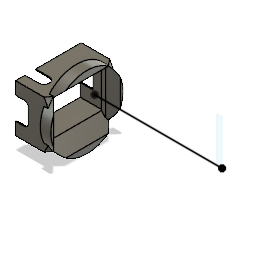
PS Vita Akaso Case v2 (Autodesk Fusion 360 design; units mm, degrees)
Autodesk Fusion 360 part; units mm, degrees
sketch "Sketch1" plane through (0, 0, 0) normal (1, 0, 0) x (0, 0, -1)
  line L0 (0, 0) -> (59, 0)
  line L1 (59, 0) -> (59, 42)
  line L2 (59, 42) -> (0, 42)
  line L3 (0, 42) -> (0, 0)
  line L4 (59, 42) -> (41.5, 42)
  line L5 (41.5, 42) -> (41.5, 24.5)
  line L6 (41.5, 24.5) -> (59, 24.5)
  line L7 (59, 24.5) -> (59, 42)
  circle A0 centre (41.5, 24.5) radius 10.5
  dimension "d1" = 59
  dimension "d2" = 42
  dimension "d3" = 17.5
  dimension "d4" = 17.5
  dimension "d5" = 21
  constraint horizontal L0
  constraint vertical L1
  constraint horizontal L2
  constraint vertical L3
  constraint coincident L0.start L3.end
  constraint horizontal L4
  constraint vertical L5
  constraint horizontal L6
  constraint vertical L7
  constraint coincident L5.end L6.start
  measures "d1" distance of L0.start L0.end
  measures "d2" distance of L0.start L2.end
  measures "d3" distance of L1.end L4.end
  measures "d4" distance of L1.end L6.end
  measures "d5" diameter of A0
extrude "Extrude1" add sketch "Sketch1" against normal blind 25 makes body 1
extrude "Extrude2" add sketch "Sketch1" along normal blind 5 contours L5 L6 A0 | L5 L6 A0 bodies 1
sketch "Sketch2" plane through (0, 0, 0) normal (1, 0, 0) x (0, 0, -1)
  line L0 (0, 0) -> (-182, 0)
  line L1 (0, 0) -> (-182, 0)
  line L2 (-182, 0) -> (-182, 84)
  line L3 (-182, 84) -> (0, 84)
  line L4 (0, 84) -> (0, 0)
  dimension "d10" = 182
  dimension "d11" = 182
  dimension "d12" = 84
  constraint coincident L0.start L1.start
  constraint horizontal L0
  constraint horizontal L1
  constraint vertical L2
  constraint horizontal L3
  constraint vertical L4
  measures "d10" distance of L0.start L0.end
  measures "d11" distance of L0.start L0.end
  measures "d12" distance of L0.start L3.end
extrude "Extrude3" add sketch "Sketch2" along normal blind 150 and the other way blind -132 separate body makes body 2
sketch "Sketch3" plane through (132, 0, 0) normal (-1, 0, 0) x (0, 0, 1)
  line L0 (182, 84) -> (0, 84)
  line L1 (0, 84) -> (0, 0)
  line L2 (0, 0) -> (182, 0)
  line L3 (182, 0) -> (182, 84)
  line L4 (0, 42) -> (182, 42)
  line L5 (91, 84) -> (91, 0)
  point P0 (0, 42)
  constraint coincident P0 L4.start
  constraint midpoint L3 L4.end
  constraint midpoint L0 L5.start
  constraint midpoint L2 L5.end
extrude "Extrude4" add sketch "Sketch3" along normal blind 5 contours L0 L3 L4 L5 bodies 2
sketch "Sketch4" plane through (0, 0, 91) normal (0, 0, -1) x (-1, 0, 0)
  line L0 (-132, 84) -> (-132, 42)
  line L1 (-132, 42) -> (-127, 42)
  line L2 (-127, 42) -> (-127, 84)
  line L3 (-127, 84) -> (-132, 84)
  line L4 (-132, 42) -> (-12, 42)
  dimension "d19" = 120
  constraint coincident L0.end L1.start
  constraint perpendicular L2 L4
  measures "d19" distance of L0.end L4.end
move_body "Move1" bodies 1 to x (1, 0, 0) y (0, 1, 0) z (0, 0, 1) at (-8.649, 1.2848, 93.06)
move_body "Move2" bodies 1 to x (1, 0, 0) y (0, 1, 0) z (0, 0, 1) at (15, 15, 40)
extrude "Extrude5" cut 1 faces at (127, 70, 121.3333) along direction (1, 0, 0) blind 5 on bodies 2 bodies 2
sketch "Sketch5" plane through (0, 0, 74.06) normal (0, 0, -1) x (-1, 0, 0)
  line L0 (-6.351, 58.2848) -> (-6.351, 16.2848)
  line L1 (-6.351, 16.2848) -> (18.649, 16.2848)
  line L2 (18.649, 16.2848) -> (18.649, 58.2848)
  line L3 (18.649, 58.2848) -> (-6.351, 58.2848)
  line L4 (-6.351, 58.2848) -> (-6.351, 58.7848)
  line L5 (-6.351, 58.7848) -> (-6.851, 58.7848)
  line L6 (-6.851, 58.7848) -> (19.149, 58.7848)
  line L7 (19.149, 58.7848) -> (19.149, 15.7848)
  line L8 (19.149, 15.7848) -> (-6.851, 15.7848)
  line L9 (-6.851, 15.7848) -> (-6.851, 58.7848)
  dimension "d22" = 0.5
  dimension "d23" = 0.5
  dimension "d24" = 43
  dimension "d25" = 26
  constraint coincident L0.start L3.end
  constraint vertical L4
  constraint perpendicular L4 L5
  constraint horizontal L6
  constraint vertical L7
  constraint horizontal L8
  constraint vertical L9
  measures "d22" distance of L0.start L4.end
  measures "d23" distance of L4.end L5.end
  measures "d24" distance of L5.end L8.end
  measures "d25" distance of L5.end L6.end
extrude "Extrude6" add sketch "Sketch5" along normal blind 2 and the other way blind -0.5 separate body makes body 3
sketch "Sketch6" plane through (0, 0, 72.06) normal (0, 0, -1) x (-1, 0, 0)
  line L0 (-6.351, 58.2848) -> (18.649, 58.2848)
  line L1 (18.649, 58.2848) -> (18.649, 16.2848)
  line L2 (18.649, 16.2848) -> (-6.351, 16.2848)
  line L3 (-6.351, 16.2848) -> (-6.351, 58.2848)
  line L4 (-6.851, 15.7848) -> (19.149, 15.7848)
  line L5 (19.149, 15.7848) -> (19.149, 58.7848)
  line L6 (19.149, 58.7848) -> (-6.851, 58.7848)
  line L7 (-6.851, 58.7848) -> (-6.851, 15.7848)
extrude "Extrude7" add sketch "Sketch6" against normal blind 0.5 contours L0 L1 L2 L3 bodies 3
extrude "Extrude8" add 1 faces at (-1.9824, 44.2848, 72.56) along direction (0, 0, 1) blind 1 on bodies 3 bodies 3
extrude "Extrude9" add 1 faces at (6.851, 30.1181, 73.06) along direction (1, 0, 0) blind 1 on bodies 3 bodies 3
sketch "Sketch7" plane through (0, 0, 73.56) normal (0, 0, 1) x (1, 0, 0)
  line L0 (-19.149, 15.7848) -> (7.851, 15.7848)
  line L1 (7.851, 15.7848) -> (7.851, 58.7848)
  line L2 (7.851, 58.7848) -> (-19.149, 58.7848)
  line L3 (-19.149, 58.7848) -> (-19.149, 15.7848)
  line L4 (7.851, 58.7848) -> (6.851, 58.7848)
  line L5 (6.851, 58.7848) -> (6.851, 15.7848)
  line L6 (6.851, 15.7848) -> (7.851, 15.7848)
  line L7 (7.851, 15.7848) -> (7.851, 58.7848)
  dimension "d36" = 1
  constraint horizontal L4
  constraint vertical L5
  constraint horizontal L6
  constraint vertical L7
  constraint coincident L1.end L2.start
  measures "d36" distance of L1.end L4.end
extrude "Extrude10" add sketch "Sketch7" along normal blind 6 contours L0 L1 L2 L4 L5 L6 L7 bodies 3
extrude "Extrude11" add 1 faces at (-1.4824, 58.7848, 72.56) along direction (0, 1, 0) blind 1 on bodies 3 bodies 3
sketch "Sketch8" plane through (0, 0, 73.56) normal (0, 0, 1) x (1, 0, 0)
  line L0 (6.851, 15.7848) -> (6.851, 59.7848)
  line L1 (6.851, 59.7848) -> (-19.149, 59.7848)
  line L2 (-19.149, 59.7848) -> (-19.149, 15.7848)
  line L3 (-19.149, 15.7848) -> (6.851, 15.7848)
  line L4 (6.851, 59.7848) -> (-19.149, 59.7848)
  line L5 (-19.149, 59.7848) -> (-19.149, 58.7848)
  line L6 (-19.149, 58.7848) -> (6.851, 58.7848)
  line L7 (6.851, 58.7848) -> (6.851, 59.7848)
  dimension "d41" = 1
  constraint horizontal L4
  constraint vertical L5
  constraint horizontal L6
  constraint vertical L7
  constraint coincident L0.end L1.start
  measures "d41" distance of L0.end L6.end
extrude "Extrude12" add sketch "Sketch8" along normal blind 61 contours L0 L1 L2 L4 L5 L6 L7 bodies 3
sketch "Sketch9" plane through (0, 58.7848, 0) normal (0, -1, 0) x (1, 0, 0)
  line L0 (-19.149, 73.56) -> (6.851, 73.56)
  line L1 (6.851, 73.56) -> (6.851, 79.56)
  line L2 (6.851, 79.56) -> (6.851, 134.56)
  line L3 (6.851, 134.56) -> (-19.149, 134.56)
  line L4 (-19.149, 134.56) -> (-19.149, 73.56)
  line L5 (-19.149, 134.56) -> (6.851, 134.56)
  line L6 (6.851, 134.56) -> (6.851, 133.56)
  line L7 (6.851, 133.56) -> (-19.149, 133.56)
  line L8 (-19.149, 133.56) -> (-19.149, 134.56)
  dimension "d44" = 1
  constraint horizontal L5
  constraint vertical L6
  constraint horizontal L7
  constraint vertical L8
  constraint coincident L3.end L4.start
  measures "d44" distance of L3.end L7.end
extrude "Extrude13" add sketch "Sketch9" along normal blind 44 contours L2 L3 L4 L5 L6 L7 L8 bodies 3
sketch "Sketch10" plane through (0, 0, 133.56) normal (0, 0, -1) x (-1, 0, 0)
  line L0 (19.149, 58.7848) -> (-6.851, 58.7848)
  line L1 (-6.851, 58.7848) -> (-6.851, 14.7848)
  line L2 (-6.851, 14.7848) -> (19.149, 14.7848)
  line L3 (19.149, 14.7848) -> (19.149, 58.7848)
  line L4 (19.149, 14.7848) -> (-6.851, 14.7848)
  line L5 (-6.851, 14.7848) -> (-6.851, 15.7848)
  line L6 (-6.851, 15.7848) -> (19.149, 15.7848)
  line L7 (19.149, 15.7848) -> (19.149, 14.7848)
  point P0 (-6.851, 15.7848)
  constraint horizontal L4
  constraint vertical L5
  constraint horizontal L6
  constraint vertical L7
  constraint coincident P0 L5.end
  constraint coincident L2.end L3.start
extrude "Extrude14" add 1 faces at (-1.4824, 15.7848, 72.56) along direction (0, -1, 0) blind 1 on bodies 3 bodies 3
extrude "Extrude15" add sketch "Sketch10" along normal blind 60 contours L1 L2 L3 L4 L5 L6 L7 bodies 3
extrude "Extrude16" add 1 faces at (6.851, 15.1181, 115.8933) along direction (1, 0, 0) blind 1 on bodies 3 bodies 3
sketch "Sketch11" plane through (0, 0, 133.56) normal (0, 0, -1) x (-1, 0, 0)
  line L0 (-7.851, 15.7848) -> (19.149, 15.7848)
  line L1 (19.149, 15.7848) -> (19.149, 58.7848)
  line L2 (19.149, 58.7848) -> (-7.851, 58.7848)
  line L3 (-7.851, 58.7848) -> (-7.851, 15.7848)
  line L4 (-7.851, 15.7848) -> (-6.851, 15.7848)
  line L5 (-6.851, 15.7848) -> (-6.851, 58.7848)
  line L6 (-6.851, 58.7848) -> (-7.851, 58.7848)
  line L7 (-7.851, 58.7848) -> (-7.851, 15.7848)
  dimension "d53" = 1
  constraint horizontal L4
  constraint vertical L5
  constraint horizontal L6
  constraint vertical L7
  constraint coincident L0.start L3.end
  measures "d53" distance of L0.start L4.end
extrude "Extrude17" add sketch "Sketch11" along normal blind 5 contours L0 L2 L3 L4 L5 L6 L7 bodies 3
sketch "Sketch12" plane through (0, 58.7848, 0) normal (0, -1, 0) x (1, 0, 0)
  line L0 (7.851, 128.56) -> (6.851, 128.56)
  line L1 (6.851, 128.56) -> (6.851, 133.56)
  line L2 (6.851, 133.56) -> (-19.149, 133.56)
  line L3 (-19.149, 133.56) -> (-19.149, 73.56)
  line L4 (-19.149, 73.56) -> (6.851, 73.56)
  line L5 (6.851, 73.56) -> (6.851, 79.56)
  line L6 (6.851, 79.56) -> (7.851, 79.56)
  line L7 (7.851, 79.56) -> (7.851, 128.56)
  line L8 (7.851, 128.56) -> (6.851, 128.56)
  line L9 (6.851, 128.56) -> (6.851, 79.56)
  line L10 (6.851, 79.56) -> (7.851, 79.56)
  line L11 (7.851, 79.56) -> (7.851, 128.56)
  constraint horizontal L8
  constraint vertical L9
  constraint horizontal L10
  constraint vertical L11
  constraint coincident L5.end L6.start
  constraint coincident L0.start L7.end
extrude "Extrude18" add sketch "Sketch12" along normal blind 5 contours L0 L6 L7 L8 L9 L10 L11 bodies 3
sketch "Sketch13" plane through (0, 15.7848, 0) normal (0, 1, 0) x (-1, 0, 0)
  line L0 (-6.851, 128.56) -> (-7.851, 128.56)
  line L1 (-7.851, 128.56) -> (-7.851, 79.56)
  line L2 (-7.851, 79.56) -> (-6.851, 79.56)
  line L3 (-6.851, 79.56) -> (-6.851, 73.56)
  line L4 (-6.851, 73.56) -> (19.149, 73.56)
  line L5 (19.149, 73.56) -> (19.149, 133.56)
  line L6 (19.149, 133.56) -> (-6.851, 133.56)
  line L7 (-6.851, 133.56) -> (-6.851, 128.56)
  line L8 (-7.851, 79.56) -> (-6.851, 79.56)
  line L9 (-6.851, 79.56) -> (-6.851, 128.56)
  line L10 (-6.851, 128.56) -> (-7.851, 128.56)
  line L11 (-7.851, 128.56) -> (-7.851, 79.56)
  constraint horizontal L8
  constraint vertical L9
  constraint horizontal L10
  constraint vertical L11
  constraint coincident L0.start L7.end
  constraint coincident L1.end L2.start
extrude "Extrude19" add sketch "Sketch13" along normal blind 5 contours L0 L1 L2 L8 L9 L10 L11 bodies 3
sketch "Sketch14" plane through (0, 59.7848, 0) normal (0, 1, 0) x (-1, 0, 0)
  line L0 (19.149, 72.06) -> (19.149, 134.56)
  line L1 (19.149, 134.56) -> (-7.851, 134.56)
  line L2 (-7.851, 134.56) -> (-7.851, 72.06)
  line L3 (-7.851, 72.06) -> (19.149, 72.06)
  line L4 (19.149, 134.56) -> (1.149, 134.56)
  line L5 (1.149, 134.56) -> (1.149, 115.56)
  line L6 (19.149, 115.56) -> (19.149, 134.56)
  circle A0 centre (6.149, 115.56) radius 5
  line L7 (6.149, 115.56) -> (6.149, 120.56)
  line L8 (6.149, 120.56) -> (19.149, 120.56)
  line L9 (19.149, 120.56) -> (19.149, 110.56)
  line L10 (19.149, 110.56) -> (6.149, 110.56)
  line L11 (6.149, 110.56) -> (6.149, 120.56)
  dimension "d60" = 18
  dimension "d61" = 19
  dimension "d62" = 10
  dimension "d63" = 10
  constraint horizontal L4
  constraint vertical L5
  constraint vertical L6
  constraint coincident L0.end L1.start
  constraint coincident L5.end A0
  constraint coincident A0.centre L7.start
  constraint coincident A0 L7.end
  constraint vertical L7
  constraint horizontal L8
  constraint vertical L9
  constraint horizontal L10
  constraint vertical L11
  measures "d60" distance of L0.end L4.end
  measures "d61" distance of L0.end L6.start
  measures "d62" diameter of A0
  measures "d63" distance of L7.end L10.end
extrude "Extrude20" cut sketch "Sketch14" against normal blind 1 contours L0 L6 A0 L8 L9 L10 | A0 L7 L11 | A0 L7 L11 bodies 3
sketch "Sketch15" plane through (0, 0, 134.56) normal (0, 0, 1) x (1, 0, 0)
  line L0 (7.851, 59.7848) -> (-19.149, 59.7848)
  line L1 (-19.149, 59.7848) -> (-19.149, 14.7848)
  line L2 (-19.149, 14.7848) -> (7.851, 14.7848)
  line L3 (7.851, 14.7848) -> (7.851, 59.7848)
  line L4 (-19.149, 59.7848) -> (-7.149, 59.7848)
  line L5 (-7.149, 59.7848) -> (-7.149, 47.7848)
  line L6 (-7.149, 47.7848) -> (-19.149, 47.7848)
  line L7 (-19.149, 47.7848) -> (-19.149, 59.7848)
  line L8 (-19.149, 14.7848) -> (-7.149, 14.7848)
  line L9 (-7.149, 14.7848) -> (-7.149, 26.7848)
  line L10 (-7.149, 26.7848) -> (-19.149, 26.7848)
  line L11 (-19.149, 26.7848) -> (-19.149, 14.7848)
  line L12 (-7.149, 26.7848) -> (-10.649, 26.7848)
  circle A0 centre (-10.649, 30.2848) radius 3.5
  line L13 (-7.149, 47.7848) -> (-10.649, 47.7848)
  circle A1 centre (-10.649, 44.2848) radius 3.5
  line L14 (-10.649, 44.2848) -> (-7.149, 44.2848)
  line L15 (-10.649, 30.2848) -> (-7.149, 30.2848)
  line L16 (-7.149, 30.2848) -> (-7.149, 44.2848)
  dimension "d66" = 12
  dimension "d67" = 12
  dimension "d68" = 12
  dimension "d69" = 12
  dimension "d70" = 3.5
  dimension "d71" = 7
  dimension "d72" = 3.5
  dimension "d73" = 7
  constraint horizontal L4
  constraint vertical L5
  constraint horizontal L6
  constraint vertical L7
  constraint coincident L0.end L1.start
  constraint horizontal L8
  constraint vertical L9
  constraint horizontal L10
  constraint vertical L11
  constraint coincident L1.end L2.start
  constraint perpendicular L9 L12
  constraint coincident L12.end A0
  constraint perpendicular L5 L13
  constraint coincident L13.end A1
  constraint coincident A1.centre L14.start
  constraint coincident A1 L14.end
  constraint horizontal L14
  constraint coincident A0.centre L15.start
  constraint coincident A0 L15.end
  constraint parallel L10 L15
  constraint tangent A1 L16
  measures "d66" distance of L0.end L6.end
  measures "d67" distance of L0.end L4.end
  measures "d68" distance of L1.end L10.end
  measures "d69" distance of L1.end L8.end
  measures "d70" distance of L9.end L12.end
  measures "d71" diameter of A0
  measures "d72" distance of L5.end L13.end
  measures "d73" diameter of A1
extrude "Extrude21" cut sketch "Sketch15" against normal blind 1 contours L1 L6 L10 A0 A1 L16 | A1 | A0 bodies 3
sketch "Sketch16" plane through (0, 0, 72.06) normal (0, 0, -1) x (-1, 0, 0)
  line L0 (19.149, 14.7848) -> (19.149, 59.7848)
  line L1 (19.149, 59.7848) -> (-7.851, 59.7848)
  line L2 (-7.851, 59.7848) -> (-7.851, 14.7848)
  line L3 (-7.851, 14.7848) -> (19.149, 14.7848)
  line L4 (19.149, 59.7848) -> (7.149, 59.7848)
  line L5 (7.149, 59.7848) -> (7.149, 48.7848)
  line L6 (7.149, 48.7848) -> (19.149, 48.7848)
  line L7 (19.149, 48.7848) -> (19.149, 59.7848)
  line L8 (7.149, 48.7848) -> (19.149, 48.7848)
  line L9 (19.149, 48.7848) -> (19.149, 27.7848)
  line L10 (19.149, 27.7848) -> (7.149, 27.7848)
  line L11 (7.149, 27.7848) -> (7.149, 48.7848)
  dimension "d76" = 11
  dimension "d77" = 12
  dimension "d78" = 21
  constraint horizontal L4
  constraint vertical L5
  constraint horizontal L6
  constraint vertical L7
  constraint coincident L0.end L1.start
  constraint horizontal L8
  constraint vertical L9
  constraint horizontal L10
  constraint vertical L11
  measures "d76" distance of L0.end L6.end
  measures "d77" distance of L0.end L4.end
  measures "d78" distance of L5.end L10.end
extrude "Extrude22" cut sketch "Sketch16" against normal blind 1 contours L0 L6 L8 L9 L10 L11 bodies 3
extrude "Extrude23" cut 1 faces at (-11.149, 41.7848, 73.06) along direction (0, 0, 1) blind 1 on bodies 3 bodies 3
extrude "Extrude24" cut 1 faces at (2.851, 34.1181, 72.06) along direction (0, 0, 1) blind 0.5 on bodies 3 bodies 3
move_face "MoveFace1" to x (1, 0, 0) y (0, 1, 0) z (0, 0, 1) at (0, 0, 5) 3 faces at (-10.4824, 59.4515, 120.56) (-1.5915, 59.1181, 117.6164) (-14.8157, 59.4515, 110.56) on bodies 3
sketch "Sketch17" plane through (132, 0, 0) normal (-1, 0, 0) x (0, 0, 1)
  line L0 (182, 0) -> (182, 84)
  line L1 (182, 84) -> (0, 84)
  line L2 (0, 84) -> (0, 0)
  line L3 (0, 0) -> (182, 0)
  line L4 (0, 0) -> (10, 0)
  line L5 (10, 0) -> (10, 40)
  line L6 (10, 40) -> (0, 40)
  line L7 (0, 40) -> (0, 0)
  dimension "d85" = 40
  dimension "d86" = 10
  constraint horizontal L4
  constraint vertical L5
  constraint horizontal L6
  constraint vertical L7
  constraint coincident L2.end L3.start
  measures "d85" distance of L2.end L6.end
  measures "d86" distance of L2.end L4.end
extrude "Extrude25" add sketch "Sketch17" along normal blind 1.5 and the other way blind -0.5 separate body contours L2 L3 L4 L5 L6 L7 makes body 4
extrude "Extrude26" add 1 faces at (131.1667, 26.6667, 0) along direction (0, 0, -1) blind 5.5 on bodies 4 bodies 4
sketch "Sketch18" plane through (131.5, 0, 0) normal (1, 0, 0) x (0, 0, -1)
  line L0 (5.5, 40) -> (-10, 40)
  line L1 (-10, 40) -> (-10, 0)
  line L2 (-10, 0) -> (5.5, 0)
  line L3 (5.5, 0) -> (5.5, 40)
  line L4 (5.5, 40) -> (0.5, 40)
  line L5 (0.5, 40) -> (0.5, 0)
  line L6 (0.5, 0) -> (5.5, 0)
  line L7 (5.5, 0) -> (5.5, 40)
  dimension "d93" = 5
  constraint horizontal L4
  constraint vertical L5
  constraint horizontal L6
  constraint vertical L7
  constraint coincident L0.start L3.end
  measures "d93" distance of L0.start L4.end
extrude "Extrude27" add sketch "Sketch18" along normal blind 19.5 contours L0 L2 L3 L4 L5 L6 L7 bodies 4
extrude "Extrude28" add 1 faces at (151, 26.6667, -3.8333) along direction (1, 0, 0) blind 0.5 on bodies 4 bodies 4
sketch "Sketch20" plane through (0, 0, -0.5) normal (0, 0, 1) x (1, 0, 0)
  line L0 (131.5, 40) -> (131.5, 0)
  line L1 (131.5, 0) -> (151.5, 0)
  line L2 (151.5, 0) -> (151.5, 40)
  line L3 (151.5, 40) -> (131.5, 40)
  line L4 (151.5, 0) -> (150.5, 0)
  line L5 (150.5, 0) -> (150.5, 40)
  line L6 (150.5, 40) -> (151.5, 40)
  line L7 (151.5, 40) -> (151.5, 0)
  dimension "d98" = 1
  constraint horizontal L4
  constraint vertical L5
  constraint horizontal L6
  constraint vertical L7
  constraint coincident L1.end L2.start
  measures "d98" distance of L1.end L4.end
extrude "Extrude29" add sketch "Sketch20" along normal blind 25 contours L1 L2 L3 L4 L5 L6 L7 bodies 4
extrude "Extrude30" add 1 faces at (130.5, 13.3333, 4.8333) along direction (-1, 0, 0) blind 1 on bodies 4 bodies 4
extrude "Extrude31" add 1 faces at (151.5, 13.3333, 4.5) along direction (1, 0, 0) blind 1 on bodies 4 bodies 4
extrude "Extrude32" add 1 faces at (137.8333, 0, -3.8333) along direction (0, -1, 0) blind 2 on bodies 4 bodies 4
sketch "Sketch21" plane through (0, 0, -0.5) normal (0, 0, 1) x (1, 0, 0)
  line L0 (150.5, -2) -> (150.5, 40)
  line L1 (150.5, 40) -> (131.5, 40)
  line L2 (131.5, 40) -> (131.5, -2)
  line L3 (131.5, -2) -> (150.5, -2)
  line L4 (150.5, -2) -> (131.5, -2)
  line L5 (131.5, -2) -> (131.5, -0.5)
  line L6 (131.5, -0.5) -> (150.5, -0.5)
  line L7 (150.5, -0.5) -> (150.5, -2)
  dimension "d107" = 1.5
  constraint horizontal L4
  constraint vertical L5
  constraint horizontal L6
  constraint vertical L7
  constraint coincident L0.start L3.end
  measures "d107" distance of L0.start L6.end
extrude "Extrude33" add sketch "Sketch21" along normal blind 182.5 contours L0 L2 L3 L4 L5 L6 L7 bodies 4
extrude "Extrude34" add 1 faces at (144.1667, -1.5, 182) along direction (0, 0, 1) blind 5.5 on bodies 4 bodies 4
sketch "Sketch22" plane through (0, -0.5, 0) normal (0, 1, 0) x (-1, 0, 0)
  line L0 (-150.5, -0.5) -> (-131.5, -0.5)
  line L1 (-131.5, -0.5) -> (-131.5, 10)
  line L2 (-131.5, 10) -> (-131.5, 187.5)
  line L3 (-131.5, 187.5) -> (-150.5, 187.5)
  line L4 (-150.5, 187.5) -> (-150.5, 24.5)
  line L5 (-150.5, 24.5) -> (-150.5, -0.5)
  line L6 (-150.5, 187.5) -> (-131.5, 187.5)
  line L7 (-131.5, 187.5) -> (-131.5, 182.5)
  line L8 (-131.5, 182.5) -> (-150.5, 182.5)
  line L9 (-150.5, 182.5) -> (-150.5, 187.5)
  dimension "d112" = 5
  constraint horizontal L6
  constraint vertical L7
  constraint horizontal L8
  constraint vertical L9
  constraint coincident L3.end L4.start
  measures "d112" distance of L3.end L8.end
extrude "Extrude35" add sketch "Sketch22" along normal blind 40 contours L2 L3 L4 L6 L7 L8 L9 bodies 4
extrude "Extrude36" add 1 faces at (144.1667, 39.5, 184.1667) along direction (0, 1, 0) blind 0.5 on bodies 4 bodies 4
sketch "Sketch23" plane through (131.5, 0, 0) normal (-1, 0, 0) x (0, 0, 1)
  line L0 (10, -0.5) -> (10, -2)
  line L1 (10, -2) -> (187.5, -2)
  line L2 (187.5, -2) -> (187.5, 40)
  line L3 (187.5, 40) -> (182.5, 40)
  line L4 (182.5, 40) -> (182.5, -0.5)
  line L5 (182.5, -0.5) -> (10, -0.5)
  line L6 (182.5, 40) -> (187.5, 40)
  line L7 (187.5, 40) -> (187.5, -2)
  line L8 (187.5, -2) -> (182.5, -2)
  line L9 (182.5, -2) -> (182.5, 40)
  constraint horizontal L6
  constraint vertical L7
  constraint horizontal L8
  constraint vertical L9
  constraint coincident L1.end L2.start
  constraint coincident L3.end L4.start
extrude "Extrude37" add sketch "Sketch23" along normal blind 2 contours L1 L2 L3 L4 L6 L7 L8 L9 bodies 4
sketch "Sketch24" plane through (150.5, 0, 0) normal (1, 0, 0) x (0, 0, -1)
  line L0 (-24.5, -2) -> (-24.5, -0.5)
  line L1 (-24.5, -0.5) -> (-182.5, -0.5)
  line L2 (-182.5, -0.5) -> (-182.5, 40)
  line L3 (-182.5, 40) -> (-187.5, 40)
  line L4 (-187.5, 40) -> (-187.5, -2)
  line L5 (-187.5, -2) -> (-24.5, -2)
  line L6 (-187.5, 40) -> (-182.5, 40)
  line L7 (-182.5, 40) -> (-182.5, -0.5)
  line L8 (-182.5, -0.5) -> (-187.5, -0.5)
  line L9 (-187.5, -0.5) -> (-187.5, 40)
  line L10 (-182.5, -0.5) -> (-187.5, -0.5)
  line L11 (-187.5, -0.5) -> (-187.5, -2)
  line L12 (-187.5, -2) -> (-182.5, -2)
  line L13 (-182.5, -2) -> (-182.5, -0.5)
  constraint horizontal L6
  constraint vertical L7
  constraint horizontal L8
  constraint vertical L9
  constraint coincident L1.end L2.start
  constraint coincident L3.end L4.start
  constraint horizontal L10
  constraint vertical L11
  constraint horizontal L12
  constraint vertical L13
  constraint coincident L4.end L5.start
extrude "Extrude38" add sketch "Sketch24" along normal blind 2 contours L4 L5 L8 L10 L11 L12 L13 | L2 L3 L4 L6 L7 L8 L9 L10 bodies 4
sketch "Sketch25" plane through (0, 0, 182.5) normal (0, 0, -1) x (-1, 0, 0)
  line L0 (-150.5, -0.5) -> (-131.5, -0.5)
  line L1 (-131.5, -0.5) -> (-131.5, -2)
  line L2 (-131.5, -2) -> (-129.5, -2)
  line L3 (-129.5, -2) -> (-129.5, 40)
  line L4 (-129.5, 40) -> (-152.5, 40)
  line L5 (-152.5, 40) -> (-152.5, -2)
  line L6 (-152.5, -2) -> (-150.5, -2)
  line L7 (-150.5, -2) -> (-150.5, -0.5)
  line L8 (-150.5, -2) -> (-152.5, -2)
  line L9 (-152.5, -2) -> (-152.5, 40)
  line L10 (-152.5, 40) -> (-150.5, 40)
  line L11 (-150.5, 40) -> (-150.5, -2)
  constraint horizontal L8
  constraint vertical L9
  constraint horizontal L10
  constraint vertical L11
  constraint coincident L4.end L5.start
  constraint coincident L6.end L7.start
extrude "Extrude39" add sketch "Sketch25" along normal blind 25 contours L4 L5 L6 L7 L8 L9 L10 L11 bodies 4
sketch "Sketch26" plane through (0, 0, 182.5) normal (0, 0, -1) x (-1, 0, 0)
  line L0 (-150.5, 40) -> (-150.5, -0.5)
  line L1 (-150.5, -0.5) -> (-131.5, -0.5)
  line L2 (-131.5, -0.5) -> (-131.5, -2)
  line L3 (-131.5, -2) -> (-129.5, -2)
  line L4 (-129.5, -2) -> (-129.5, 40)
  line L5 (-129.5, 40) -> (-150.5, 40)
  line L6 (-131.5, -2) -> (-129.5, -2)
  line L7 (-129.5, -2) -> (-129.5, 40)
  line L8 (-129.5, 40) -> (-131.5, 40)
  line L9 (-131.5, 40) -> (-131.5, -2)
  constraint horizontal L6
  constraint vertical L7
  constraint horizontal L8
  constraint vertical L9
  constraint coincident L4.end L5.start
  constraint coincident L2.end L3.start
extrude "Extrude40" add sketch "Sketch26" along normal blind 10 contours L2 L3 L4 L5 L6 L7 L8 L9 bodies 4
extrude "Extrude41" add 1 faces at (131.5, -1, 118.3333) along direction (-1, 0, 0) blind 2 on bodies 4 bodies 4
sketch "Sketch27" plane through (0, -0.5, 0) normal (0, 1, 0) x (-1, 0, 0)
  line L0 (-131.5, 182.5) -> (-150.5, 182.5)
  line L1 (-150.5, 182.5) -> (-150.5, 157.5)
  line L2 (-150.5, 157.5) -> (-150.5, 24.5)
  line L3 (-150.5, 24.5) -> (-150.5, -0.5)
  line L4 (-150.5, -0.5) -> (-131.5, -0.5)
  line L5 (-131.5, -0.5) -> (-131.5, 10)
  line L6 (-131.5, 10) -> (-129.5, 10)
  line L7 (-129.5, 10) -> (-129.5, 172.5)
  line L8 (-129.5, 172.5) -> (-131.5, 172.5)
  line L9 (-131.5, 172.5) -> (-131.5, 182.5)
  line L10 (-129.5, 10) -> (-131.5, 10)
  line L11 (-131.5, 10) -> (-131.5, 172.5)
  line L12 (-131.5, 172.5) -> (-129.5, 172.5)
  line L13 (-129.5, 172.5) -> (-129.5, 10)
  constraint horizontal L10
  constraint vertical L11
  constraint horizontal L12
  constraint vertical L13
  constraint coincident L8.end L9.start
  constraint coincident L6.end L7.start
extrude "Extrude42" add sketch "Sketch27" along normal blind 10 contours L6 L7 L8 L10 L11 L12 L13 bodies 4
extrude "Extrude43" add 1 faces at (150.5, -1.5, 113.1667) along direction (1, 0, 0) blind 2 on bodies 4 bodies 4
sketch "Sketch28" plane through (0, -0.5, 0) normal (0, 1, 0) x (-1, 0, 0)
  line L0 (-131.5, -0.5) -> (-131.5, 182.5)
  line L1 (-131.5, 182.5) -> (-150.5, 182.5)
  line L2 (-150.5, 182.5) -> (-150.5, 157.5)
  line L3 (-150.5, 157.5) -> (-152.5, 157.5)
  line L4 (-152.5, 157.5) -> (-152.5, 24.5)
  line L5 (-152.5, 24.5) -> (-150.5, 24.5)
  line L6 (-150.5, 24.5) -> (-150.5, -0.5)
  line L7 (-150.5, -0.5) -> (-131.5, -0.5)
  line L8 (-152.5, 157.5) -> (-150.5, 157.5)
  line L9 (-150.5, 157.5) -> (-150.5, 24.5)
  line L10 (-150.5, 24.5) -> (-152.5, 24.5)
  line L11 (-152.5, 24.5) -> (-152.5, 157.5)
  constraint horizontal L8
  constraint vertical L9
  constraint horizontal L10
  constraint vertical L11
  constraint coincident L5.end L6.start
  constraint coincident L3.end L4.start
extrude "Extrude44" add sketch "Sketch28" along normal blind 35 contours L3 L4 L5 L8 L9 L10 L11 bodies 4
sketch "Sketch29" plane through (7.851, 0, 0) normal (1, 0, 0) x (0, 0, -1)
  line L0 (-72.56, 14.7848) -> (-72.56, 59.7848)
  line L1 (-72.56, 59.7848) -> (-134.56, 59.7848)
  line L2 (-134.56, 59.7848) -> (-134.56, 14.7848)
  line L3 (-134.56, 14.7848) -> (-72.56, 14.7848)
  line L4 (-79.56, 53.7848) -> (-79.56, 20.7848)
  line L5 (-79.56, 20.7848) -> (-128.56, 20.7848)
  line L6 (-128.56, 20.7848) -> (-128.56, 53.7848)
  line L7 (-128.56, 53.7848) -> (-79.56, 53.7848)
  line L8 (-128.56, 37.2848) -> (-79.56, 37.2848)
  circle A0 centre (-104.06, 37.2848) radius 34
  dimension "d133" = 68
  constraint midpoint L6 L8.start
  constraint midpoint L4 L8.end
  constraint midpoint L8 A0.centre
  measures "d133" diameter of A0
extrude "Extrude45" add sketch "Sketch29" along normal blind 10 contours L0 L1 L2 L3 A0 | L0 A0 | L3 A0 | L1 A0 | L2 A0 bodies 3
chamfer "Chamfer1" distance 3.9 angle 45 1 edges at (7.851, 56.2138, 132.3034) on bodies 3
chamfer "Chamfer2" distance 3.9 angle 45 1 edges at (7.851, 18.3558, 132.3034) on bodies 3
chamfer "Chamfer3" distance 4.6 angle 45 1 edges at (7.851, 55.187, 75.1548) on bodies 3
chamfer "Chamfer4" distance 4.6 angle 45 1 edges at (7.851, 19.3826, 75.1548) on bodies 3
chamfer "Chamfer5" distance 11 angle 45 1 edges at (17.851, 53.7848, 104.06) on bodies 3
chamfer "Chamfer6" distance 10.99 angle 45 1 edges at (17.851, 20.7848, 104.06) on bodies 3
chamfer "Chamfer7" distance 7 angle 45 1 edges at (17.851, 37.2848, 79.56) on bodies 3
chamfer "Chamfer8" distance 7 angle 45 1 edges at (17.851, 37.2848, 128.56) on bodies 3
hidden bodies 1 2 4
